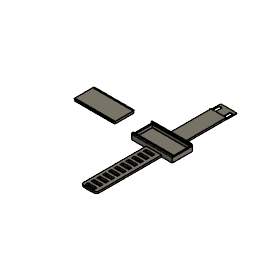
wristband and components (Autodesk Fusion 360 design; units mm, degrees)
part number: 2026-09-04-15-34-31-389
Autodesk Fusion 360 part; units mm, degrees
sketch "Sketch2" plane through (0, 0, 0) normal (0, 1, 0) x (1, 0, 0)
  line L0 (0, 0) -> (69.9996, 0)
  line L1 (69.9996, 0) -> (69.9996, 35)
  line L2 (69.9996, 35) -> (0, 35)
  line L3 (0, 35) -> (0, 0)
  dimension "d4" = 35
  constraint horizontal L0
  constraint vertical L1
  constraint horizontal L2
  constraint vertical L3
  constraint coincident L0.start L3.end
  measures "d4" distance of L0.start L2.end
extrude "Extrude2" add sketch "Sketch2" along normal blind 8 makes body 1
sketch "Sketch6" plane through (0, 0, 0) normal (0, 1, 0) x (1, 0, 0)
  line L0 (2.5, 2.5, 8) -> (68, 2.5, 8)
  line L1 (68, 2.5, 8) -> (68, 33, 8)
  line L2 (68, 33, 8) -> (2.5, 33, 8)
  line L3 (2.5, 33, 8) -> (2.5, 2.5, 8)
extrude "Extrude5" cut sketch "Sketch6" against normal blind 5 contours L0 L1 L2 L3 in plane through (0, 8, 0) normal (0, 1, 0) bodies 1
sketch "Sketch7" plane through (0, 0, 0) normal (1, 0, 0) x (0, 0, -1)
  line L0 (0, 8) -> (0, 11)
  line L1 (0, 11) -> (2, 11)
  line L2 (35, 8) -> (35, 11)
  line L3 (35, 11) -> (33, 11)
  line L4 (2, 11) -> (0.5, 8)
  line L5 (0.5, 8) -> (0, 8)
  line L6 (33, 11) -> (34.5, 8)
  line L7 (34.5, 8) -> (35, 8)
  constraint vertical L0
  constraint perpendicular L0 L1
  constraint perpendicular L1 L2
  constraint perpendicular L0 L3
extrude "Extrude7" add sketch "Sketch7" along normal blind 70 bodies 1
sketch "Sketch8" plane through (0, 0, 0) normal (1, 0, 0) x (0, 0, -1)
  line L0 (0.7, 8) -> (2.2, 11)
  line L1 (34, 8) -> (0.7, 8)
  line L2 (2.2, 11) -> (2, 11.1)
  line L3 (2, 11.1) -> (0, 11.1)
  line L4 (0, 11.1) -> (0, 11.7)
  line L5 (0, 11.7) -> (35, 11.7)
  line L6 (35, 11.7) -> (35, 11.1)
  line L7 (35, 11.1) -> (33, 11.1)
  line L8 (2.2, 11) -> (32.9, 11)
  line L9 (32.9, 11) -> (34.4, 8)
  line L10 (34.4, 8) -> (34, 8)
  line L11 (33, 11.1) -> (32.9, 11)
  constraint perpendicular L0 L2
  constraint perpendicular L3 L4
  constraint perpendicular L4 L5
  constraint perpendicular L5 L6
  constraint perpendicular L6 L7
  constraint parallel L7 L8
extrude "Extrude8" add sketch "Sketch8" against normal blind 70 separate body makes body 2
move_body "Move3" bodies 2 to x (1, 0, 0) y (0, 1, 0) z (0, 0, 1) at (-30, 0, 0)
sketch "Sketch9" plane through (0, 0, 0) normal (0, 1, 0) x (1, 0, 0)
  line L0 (25, 0) -> (51.5435, 0)
  line L1 (51.5435, 0) -> (51.5435, -112.73)
  line L2 (51.5435, -112.73) -> (25, -112.73)
  line L3 (25, -112.73) -> (25, 0)
  dimension "d25" = 112.73
  constraint horizontal L0
  constraint vertical L1
  constraint horizontal L2
  constraint vertical L3
  measures "d25" distance of L0.start L2.end
extrude "Extrude9" add sketch "Sketch9" along normal blind 3 separate body makes body 3
sketch "Sketch10" plane through (0, 3, 0) normal (0, 1, 0) x (-1, 0, 0)
  line L0 (-25, 112.73) -> (-51.5435, 112.73)
  line L1 (-51.5435, 112.73) -> (-51.5435, 0)
  line L2 (-25, 0) -> (-25, 112.73)
  line L3 (-30, 5) -> (-45, 5)
  line L4 (-45, 5) -> (-45, 10)
  line L5 (-45, 10) -> (-30, 10)
  line L6 (-30, 10) -> (-30, 5)
  line L7 (-30, 15) -> (-45, 15)
  line L8 (-45, 15) -> (-45, 20)
  line L9 (-45, 20) -> (-30, 20)
  line L10 (-30, 20) -> (-30, 15)
  line L11 (-45, 25) -> (-30, 25)
  line L12 (-30, 25) -> (-30, 30)
  line L13 (-30, 30) -> (-45, 30)
  line L14 (-45, 30) -> (-45, 25)
  line L15 (-45, 35) -> (-30, 35)
  line L16 (-30, 35) -> (-30, 40)
  line L17 (-30, 40) -> (-45, 40)
  line L18 (-45, 40) -> (-45, 35)
  line L19 (-45, 45) -> (-30, 45)
  line L20 (-30, 45) -> (-30, 50)
  line L21 (-30, 50) -> (-45, 50)
  line L22 (-45, 50) -> (-45, 45)
  line L23 (-45, 55) -> (-30, 55)
  line L24 (-30, 55) -> (-30, 60)
  line L25 (-30, 60) -> (-45, 60)
  line L26 (-45, 60) -> (-45, 55)
  line L27 (-45, 65) -> (-30, 65)
  line L28 (-30, 65) -> (-30, 70)
  line L29 (-30, 70) -> (-45, 70)
  line L30 (-45, 70) -> (-45, 65)
  line L31 (-45, 75) -> (-30, 75)
  line L32 (-30, 75) -> (-30, 80)
  line L33 (-30, 80) -> (-45, 80)
  line L34 (-45, 80) -> (-45, 75)
  line L35 (-45, 85) -> (-30, 85)
  line L36 (-30, 85) -> (-30, 90)
  line L37 (-30, 90) -> (-45, 90)
  line L38 (-45, 90) -> (-45, 85)
  line L39 (-45, 95) -> (-30, 95)
  line L40 (-30, 95) -> (-30, 100)
  line L41 (-30, 100) -> (-45, 100)
  line L42 (-45, 100) -> (-45, 95)
  line L43 (-45, 105) -> (-30, 105)
  line L44 (-30, 105) -> (-30, 110)
  line L45 (-30, 110) -> (-45, 110)
  line L46 (-45, 110) -> (-45, 105)
  arc A0 (-25, 110) -> (-30, 112.5) centre (-29.75, 106.75) ccw
  line L47 (-25, 110) -> (-25, 112.73)
  line L48 (-30, 112.73) -> (-30, 112.5)
  arc A1 (-45.0416, 112.73) -> (-51.5435, 109.9998) centre (-45.0416, 103.6228) ccw
  line L49 (-51.5435, 109.9998) -> (-51.5435, 112.73)
  line L50 (-51.5435, 0) -> (-25, 0)
  constraint perpendicular L2 L3
  constraint perpendicular L3 L4
  constraint perpendicular L2 L5
  constraint perpendicular L3 L6
  constraint perpendicular L6 L7
  constraint perpendicular L7 L8
  constraint perpendicular L8 L9
  constraint perpendicular L7 L10
  constraint perpendicular L10 L11
  constraint perpendicular L11 L12
  constraint perpendicular L12 L13
  constraint perpendicular L11 L14
  constraint perpendicular L12 L15
  constraint perpendicular L15 L16
  constraint perpendicular L16 L17
  constraint perpendicular L15 L18
  constraint perpendicular L18 L19
  constraint perpendicular L17 L20
  constraint perpendicular L20 L21
  constraint perpendicular L19 L22
  constraint perpendicular L22 L23
  constraint perpendicular L21 L24
  constraint perpendicular L24 L25
  constraint perpendicular L23 L26
  constraint perpendicular L26 L27
  constraint perpendicular L27 L28
  constraint perpendicular L28 L29
  constraint perpendicular L27 L30
  constraint perpendicular L30 L31
  constraint perpendicular L31 L32
  constraint perpendicular L32 L33
  constraint perpendicular L31 L34
  constraint perpendicular L34 L35
  constraint perpendicular L35 L36
  constraint perpendicular L36 L37
  constraint perpendicular L35 L38
  constraint perpendicular L38 L39
  constraint perpendicular L39 L40
  constraint perpendicular L40 L41
  constraint perpendicular L39 L42
  constraint perpendicular L42 L43
  constraint perpendicular L43 L44
  constraint perpendicular L44 L45
  constraint perpendicular L43 L46
  constraint coincident L2 A0.start
  constraint coincident L0.start L2.end
  constraint coincident L0 L48.start
  constraint perpendicular L0 L48
  constraint tangent L0 A1
  constraint coincident L0 A1.start
  constraint coincident L1 A1.end
  constraint coincident L0.end L1.start
extrude "Extrude11" cut sketch "Sketch10" against normal blind 10 contours L0 L2 A0 L47 L48 | L0 L1 A1 L49 | L3 L4 L5 L6 | L7 L8 L9 L10 | L11 L12 L13 L14 | L15 L16 L17 L18 | L19 L20 L21 L22 | L23 L24 L25 L26 | L27 L28 L29 L30 | L31 L32 L33 L34 | L35 L36 L37 L38 | L39 L40 L41 L42 | L43 L44 L45 L46 bodies 3
sketch "Sketch12" plane through (0, 0, 0) normal (0, 1, 0) x (1, 0, 0)
  line L0 (25, 35) -> (51.543, 35)
  line L1 (51.543, 35) -> (51.543, 110)
  line L2 (51.543, 110) -> (25, 110)
  line L3 (25, 110) -> (25, 35)
  dimension "d32" = 26.543
  dimension "d33" = 26.543
  constraint horizontal L0
  constraint perpendicular L0 L1
  constraint perpendicular L1 L2
  measures "d32" distance of L0.start L0.end
  measures "d33" distance of L1.end L2.end
extrude "Extrude12" add sketch "Sketch12" along normal blind 3 separate body makes body 4
sketch "Sketch14" plane through (0, 0, 0) normal (0, 1, 0) x (1, 0, 0)
  line L0 (25, 110) -> (24, 110)
  line L1 (24, 110) -> (24, 130)
  line L2 (24, 130) -> (52, 130)
  line L3 (52, 130) -> (52, 110)
  line L4 (52, 110) -> (25, 110)
  line L5 (52, 112) -> (24, 112)
  constraint horizontal L0
  constraint perpendicular L0 L1
  constraint perpendicular L1 L2
  constraint perpendicular L0 L3
  constraint perpendicular L3 L4
  constraint coincident L3 L5.start
  constraint coincident L1 L5.end
  constraint perpendicular L1 L5
extrude "Extrude13" add sketch "Sketch14" along normal blind 3 contours L0 L1 L3 L4 L5 bodies 1 4 3
extrude "Extrude14" add sketch "Sketch14" along normal blind 1 separate body contours L1 L2 L3 L5 makes body 5
sketch "Sketch17" plane through (0, 1, 0) normal (0, 1, 0) x (-1, 0, 0)
  line L0 (-52, -112) -> (-52, -130)
  line L1 (-52, -130) -> (-24, -130)
  line L2 (-24, -130) -> (-24, -112)
  line L3 (-24, -112) -> (-52, -112)
  line L4 (-50, -112) -> (-45, -112)
  line L5 (-45, -112) -> (-45, -125)
  line L6 (-45, -125) -> (-50, -125)
  line L7 (-50, -125) -> (-50, -112)
  line L8 (-26, -112) -> (-31, -112)
  line L9 (-31, -112) -> (-31, -125)
  line L10 (-31, -125) -> (-26, -125)
  line L11 (-26, -125) -> (-26, -112)
  constraint horizontal L4
  constraint vertical L5
  constraint horizontal L6
  constraint vertical L7
  constraint coincident L3 L4.start
  constraint horizontal L8
  constraint vertical L9
  constraint horizontal L10
  constraint vertical L11
  constraint coincident L3 L8.start
extrude "Extrude15" cut sketch "Sketch17" against normal blind 180 contours L3 L4 L5 L6 L7 | L3 L8 L9 L10 L11 bodies 5
